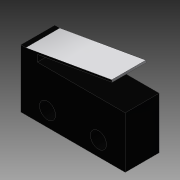
# Autodesk Inventor part: E-Stop_Zippy
Saved by Autodesk Inventor 2015 (Build 190159000, 159)
## iProperties
Created: 2015-01-06
Part Number: E-Stop_Zippy
Material: Generic
Document SubType Name: Modeling
Designer: Drew
Density: 1 g/cm^3
Appearance: Anodized - Black
Author: Drew
Autodesk Inventor part; units mm, degrees
ref_plane "YZ Plane" through (0, 0, 0) normal (1, 0, 0) x (0, 1, 0)
ref_plane "XZ Plane" through (0, 0, 0) normal (0, 1, 0) x (-1, 0, 0)
ref_plane "XY Plane" through (0, 0, 0) normal (0, 0, 1) x (1, 0, 0)
sketch "Sketch1" plane through (0, 0, 0) normal (0, 0, 1) x (1, 0, 0)
  line L0 (-9.906, -4.8895) -> (-9.906, 4.8895)
  line L1 (-6.7578, 4.8895) -> (9.906, 4.8895)
  line L2 (9.906, 4.8895) -> (9.906, -4.8895)
  line L3 (9.906, -4.8895) -> (-9.906, 4.8895) construction
  line L4 (-9.906, -4.8895) -> (9.906, 4.8895) construction
  line L5 (0, 15.8436) -> (0, -13.7401)
  line L6 (9.906, -4.8895) -> (-9.906, 4.8895) construction
  line L7 (9.906, -4.8895) -> (-9.906, -4.8895)
  line L8 (9.906, -4.8895) -> (8.255, -4.8895)
  line L9 (-9.906, 4.8895) -> (-9.906, 6.1595)
  line L10 (-9.906, 6.1595) -> (-8.9519, 6.1595)
  line L11 (-8.9519, 6.1595) -> (7.3517, 9.0343)
  line L12 (7.3517, 9.0343) -> (7.4178, 8.659)
  line L13 (7.4178, 8.659) -> (-6.7578, 6.1595)
  line L14 (-6.7578, 6.1595) -> (-6.7578, 4.8895)
  line L15 (7.4467, -4.8895) -> (0.4041, -4.8895)
  line L16 (-0.4041, -4.8895) -> (-9.906, -4.8895)
  circle A0 centre (-4.826, -2.0955) radius 1.524
  circle A1 centre (4.826, -2.0955) radius 1.524
  point P0 (0, 0)
  point P1 (-8.255, -4.8895)
  point P2 (-7.4467, -4.8895)
  point P3 (0, 0)
  point P4 (0, -9.5177)
  dimension "d4" = 9.779
  dimension "d7" = 0.381
  dimension "d8" = 10
  dimension "d9" = 19.812
  dimension "d11" = 11.049
  dimension "d16" = 3.048
  dimension "d17" = 9.652
  dimension "d18" = 2.794
  constraints: 34 end point, 8 perpendicular, 6 parallel, 6 point on line, 4 horizontal, 3 midpoint, 3 symmetric about line, 2 centre point, 1 collinear, 1 vertical, 1 other
  measures "d4" distance between parallel lines of L8 L1
  measures "d7" distance between parallel lines of L13 L11
  measures "d8" angle of L1 L13
  measures "d9" distance between parallel lines of L2 L0
  measures "d11" distance between parallel lines of L7 L10
  measures "d16" diameter of A0
  measures "d17" distance of A1.centre A0.centre
  measures "d18" distance from line of L16 A0.centre
extrude "Extrusion1" add sketch "Sketch1" along normal blind 6.4516 contours L0 L9 L10 L11 L5 L13 L14 L1 L7 | L5 L1 L2 L7 | L11 L12 L13 L5
body "Solid1"
